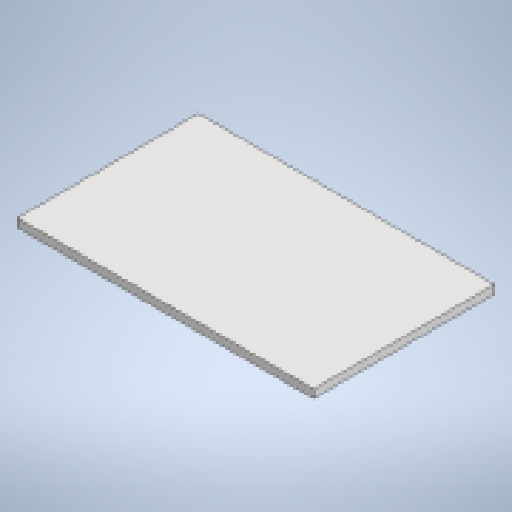
# Autodesk Inventor part: electronics plate
Saved by Autodesk Inventor 2023 (Build 270158000, 158)
## iProperties
Created: 2023-04-08
Part Number: electronics plate
Material: Generic
Document SubType Name: Modeling
Designer: ASARe-DAQ-PC
Density: 1 g/cm^3
Appearance: Default
Author: ASARe-DAQ-PC
Autodesk Inventor part; units mm, degrees
ref_plane "YZ Plane" through (0, 0, 0) normal (1, 0, 0) x (0, 1, 0)
ref_plane "XZ Plane" through (0, 0, 0) normal (0, 1, 0) x (-1, 0, 0)
ref_plane "XY Plane" through (0, 0, 0) normal (0, 0, 1) x (1, 0, 0)
sketch "Sketch1" plane through (0, 0, 0) normal (0, 1, 0) x (-1, 0, 0)
  line L0 (0, 0) -> (180, 0)
  line L1 (180, 0) -> (180, -110)
  line L2 (180, -110) -> (0, -110)
  line L3 (0, -110) -> (0, 0)
  dimension "d0" = 110
  dimension "d32" = 180
  constraints: 8 end point, 2 parallel, 1 horizontal, 1 perpendicular
  measures "d0" distance of L0.end L1.end
  measures "d32" distance of L0.start L0.end
extrude "Extrusion1" add sketch "Sketch1" against normal blind 5
body "Solid1"
